indexproximalphalanx (Autodesk Fusion 360 design; units mm, degrees)
Autodesk Fusion 360 part; units mm, degrees
sketch "Sketch1" plane through (0, 0, 0) normal (0, 0, 1) x (1, 0, 0)
  line L0 (14, 5) -> (-14, 5)
  line L1 (-14, 5) -> (-14, -5)
  line L2 (-14, -5) -> (14, -5)
  line L3 (14, -5) -> (14, 5)
  line L4 (14, 5) -> (-14, -5) construction
  line L5 (-14, 5) -> (14, -5) construction
  circle A0 centre (14, 0) radius 5
  circle A1 centre (-21.5, 0) radius 10
  circle A2 centre (15.6583, 2.5) radius 0.75
  line L6 (-14, 5) -> (14, 5)
  line L7 (14, 5) -> (14, 6)
  line L8 (14, 6) -> (-14, 6)
  line L9 (-14, 6) -> (-14, 5)
  circle A3 centre (-21.5, 0) radius 5
  line L10 (9, 0) -> (9, 5)
  line L11 (9, 0) -> (9, -5)
  circle A4 centre (14, 0) radius 0.85
  line L12 (-8.5, -1.75) -> (4.5, -1.75)
  arc A5 (4.5, -1.75) -> (4.5, 1.75) centre (4.5, 0) ccw
  line L13 (4.5, 1.75) -> (-8.5, 1.75)
  arc A6 (-8.5, 1.75) -> (-8.5, -1.75) centre (-8.5, 0) ccw
  line L14 (-8.5, 0) -> (4.5, 0) construction
  circle A7 centre (15.6583, 2.5) radius 1.5
  spline S0 degree 5 poles (15.265, 4.8373) (15.1458, 4.8016) (14.9167, 4.7248) (14.6006, 4.5934) (14.2349, 4.3855) (13.8708, 4.0716) (13.5978, 3.7066) (13.4107, 3.2967) (13.2986, 2.8544) (13.2438, 2.3979) (13.2247, 1.9423) (13.2176, 1.4913) (13.1992, 1.0293) (13.1491, 0.5092) (13.057, -0.0729) (12.9192, -0.7014) (12.7368, -1.3443) (12.5136, -1.9652) (12.2541, -2.5307) (11.9618, -3.0199) (11.639, -3.4214) (11.3576, -3.6686) (11.1337, -3.8121) (10.9789, -3.8891) (10.9, -3.923) knots 0 0 0 0 0 0 0.05 0.1 0.15 0.2 0.25 0.3 0.35 0.4 0.45 0.5 0.55 0.6 0.65 0.7 0.75 0.8 0.85 0.9 0.95 1 1 1 1 1 1
  line L15 (10.9, -3.923) -> (10.9, -5)
  circle A8 centre (-21.5, 0) radius 10.5
  line L16 (13.25, 2.2366) -> (13.1645, 0.3413)
  point P0 (13.4583, 3.3661)
  point P1 (13.2073, 1.289)
  point P2 (12.5, -1.9625)
  dimension "d1" = 28
  dimension "d2" = 10
  dimension "d6" = 20
  dimension "d7" = 7.5
  dimension "d8" = 5
  dimension "d9" = 1.5
  dimension "d10" = 3
  dimension "d12" = 2.5
  dimension "d13" = 28
  dimension "d14" = 1
  dimension "d15" = 10
  dimension "d31" = 1.7
  dimension "d35" = 3.5
  dimension "d36" = 3.25
  dimension "d47" = 3
  dimension "d57" = 21
  dimension "d79" = 2.2
  dimension "d80" = 0.75
  dimension "d81" = 1.5
  dimension "d82" = 1.265
  dimension "d83" = 3.1
  dimension "d84" = 4.5
  dimension "d85" = 13
  constraint horizontal L0
  constraint perpendicular L0 L1
  constraint parallel L0 L2
  constraint parallel L1 L3
  constraint coincident L4 origin
  constraint coincident L5 origin
  constraint midpoint L3 A0.centre
  constraint coincident L2.end A0
  constraint horizontal L6
  constraint vertical L7
  constraint horizontal L8
  constraint vertical L9
  constraint concentric A1 A3
  constraint coincident A0 L10.start
  constraint coincident L0 L10.end
  constraint tangent A0 L10
  constraint perpendicular L0 L10
  constraint coincident L2 L11.end
  constraint tangent A0 L11
  constraint concentric A0 A4
  constraint tangent L12 A5
  constraint tangent A5 L13
  constraint parallel L12 L13
  constraint tangent L13 A6
  constraint tangent L12 A6
  constraint perpendicular L10 L14
  constraint concentric A2 A7
  constraint coincident A0 S0.start
  constraint coincident A0 S0.end
  constraint coincident L2 L15.end
  constraint perpendicular L2 L15
  constraint concentric A1 A8
  constraint midpoint P1 L16
  constraint tangent A4 L16
  measures "d1" distance of L1.end L2.end
  measures "d2" distance of L0.end L1.end
  measures "d6" diameter of A1
  measures "d7" distance of L1 A1.centre
  measures "d8" distance of L2 A1.centre
  measures "d9" diameter of A2
  measures "d10" distance of A0.centre A2.centre
  measures "d12" vertical distance of A0.centre A2.centre
  measures "d13" distance of L0.end L0.start
  measures "d14" distance of L0.end L8.end
  measures "d15" diameter of A3
  measures "d31" diameter of A4
  measures "d35" diameter of A5
  measures "d36" distance of L0 L13
  measures "d47" diameter of A7
  measures "d57" diameter of A8
  measures "d79" horizontal distance of A2.centre P0
  measures "d80" distance of L3 L16.start
  measures "d81" distance of L3 P2
  measures "d82" distance of L3 S0.start
  measures "d83" distance of L3 S0.end
  measures "d84" distance of L11 A5.centre
  measures "d85" distance of A1.centre A6.centre
extrude "Extrude1" add sketch "Sketch1" along normal blind 3 contours L0 A0 L6 L10 | L3 A0 S0 | L3 A0 S0 | L0 L6 L7 L8 A8 | L0 L2 L6 L10 L11 A8 | L3 A0 A4 S0 | L3 A0 A4 S0 | L2 A0 L11 L15 | L0 L2 A1 L6 A8 | L0 A1 L6 L8 A8 | L3 A4 | L3 A4 | L2 A0 L15 | L0 L1 L2 A1 L6 | L0 A1 L6 L8 L9 | L1 L2 A1 L8 L9 | A2 | L12 A5 L13 A6 | A7
extrude "Extrude2" cut sketch "Sketch1" along normal blind 1.5 contours L3 A0 S0 | L3 A0 S0 | L3 A0 A4 S0 | L3 A0 A4 S0 | L3 A4 | L3 A4 | A7
extrude "Extrude3" cut sketch "Sketch1" along normal blind 1.5 contours L2 A0 L11 L15 | L2 A0 L15
extrude "Extrude4" cut sketch "Sketch1" along normal blind 1.5 contours A2
extrude "Extrude5" add sketch "Sketch1" along normal blind 7 contours A2
extrude "Extrude6" cut sketch "Sketch1" along normal blind 1.5 contours A2
extrude "Extrude7" add sketch "Sketch1" along normal blind 1.5 contours L3 A4 | L3 A4
ref_plane "WorkPlane1" through (-6.4638, 0.2545, 5) normal (0, 0, 1) x (1, 0, 0)
mirror "Mirror1" about plane through (-6.4638, 0.2545, 5) normal (0, 0, 1) of bodies 1 merged
extrude "Extrude8" add sketch "Sketch1" along normal blind 7 contours L0 A0 L6 L10 | L0 L6 L7 L8 A8 | L0 L2 L6 L10 L11 A8 | L0 L2 A1 L6 A8 | L0 A1 L6 L8 A8
extrude "Extrude9" cut sketch "Sketch1" along normal blind 15 contours L12 A5 L13 A6
fillet "Fillet2" radius 10 4 edges at (-12.8397, -5, 8.5) (-12.8397, -5, 1.5) (-13.5, 6, 8.5) (-13.5, 6, 1.5)
extrude "Extrude10" add sketch "Sketch1" along normal blind 4 from surface at 3 contours L3 A0 S0 | L3 A0 S0 | L2 A0 L11 L15
fillet "Fillet3" radius 10 1 edges at (10.9, -3.923, 5)
fillet "Fillet5" radius 8 2 edges at (9, -5, 9.25) (9, -5, 0.75)
extrude "Extrude11" cut sketch "Sketch1" along normal blind 7 contours L0 L2 A1 L6 A8
extrude "Extrude12" add sketch "Sketch1" along normal blind 3 contours L0 L2 A1 L6 A8
extrude "Extrude13" cut sketch "Sketch1" along normal blind 7 contours L0 A1 L6 L8 L9
extrude "Extrude14" cut sketch "Sketch1" along normal blind 7 contours L0 A1 L6 L8 A8
extrude "Extrude15" add sketch "Sketch1" along normal blind 3 contours L0 A1 L6 L8 A8 | L0 A1 L6 L8 L9
fillet "Fillet8" radius 1 14 edges at (2.25, 6, 10) (-12.6623, 6.5132, 10) (-31.4922, -0.3961, 10) (-11.8068, -5.6459, 10) (-3.4602, -5, 10) (6.3123, -3.2757, 10) (10.8991, 3.9223, 10) (2.25, 6, 0) (-12.6623, 6.5132, 0) (-31.4922, -0.3961, 0) (-11.8068, -5.6459, 0) (-3.4602, -5, 0) (6.3123, -3.2757, 0) (10.8991, 3.9223, 0)
move_face "OffsetFaces1" [suppressed]
move_face "OffsetFaces2" [suppressed]
move_face "OffsetFaces3" [suppressed]
move_face "OffsetFaces4" [suppressed]
move_face "OffsetFaces5" [suppressed]
move_face "OffsetFaces6" [suppressed]
move_face "OffsetFaces7" [suppressed]
delete_face "DeleteFace1" [suppressed]
fillet "Fillet6" [suppressed]
fillet "Fillet7" [suppressed]
equation "d1 = length"
equation "d2 = thickness"
equation "length = 28 mm"
equation "thickness = 10 mm"
equation "gap = 0.3 mm"
equation "d13 = length"
equation "d31 = 2 mm - gap"
equation "d69 = -gap"
equation "d70 = -gap"
equation "d71 = -gap"
equation "d72 = -gap"
equation "d73 = -gap"
equation "d74 = -gap"
